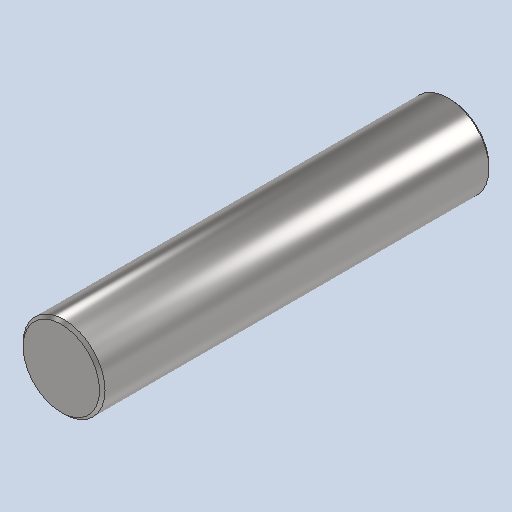
# Autodesk Inventor part: Schaft_6mmx28.5
Saved by Autodesk Inventor 2022 (Build 260153000, 153)
## iProperties
Created: 2022-10-05
Part Number: Schaft_6mmx28.5
Material: Edelstahl
Document SubType Name: Modeling
Designer: alexw
Mass: 6.44065 g
Surface Area: 5.8924 cm^2
Volume: 0.805081 cm^3
Density: 8 g/cm^3
Appearance: Halbpoliert
Author: alexw
Autodesk Inventor part; units mm, degrees
ref_plane "YZ Plane" through (0, 0, 0) normal (1, 0, 0) x (0, 1, 0)
ref_plane "XZ Plane" through (0, 0, 0) normal (0, 1, 0) x (-1, 0, 0)
ref_plane "XY Plane" through (0, 0, 0) normal (0, 0, 1) x (1, 0, 0)
sketch "Skizze1" plane through (0, 0, 0) normal (0, 0, 1) x (1, 0, 0)
  circle A0 centre (0, 0) radius 3
  dimension "d0" = 6
  constraints: 1 centre point, 1 coincident
  measures "d0" diameter of A0
extrude "Extrusion1" add sketch "Skizze1" along normal blind 28.5
chamfer "Fase1" distance 0.2 angle 45 2 edges at (-3, 0, 28.5) (-3, 0, 0)
